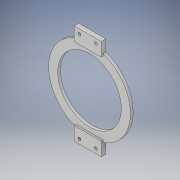
# Autodesk Inventor part: LED_Ring
Saved by Autodesk Inventor 2017 (Build 210142000, 142)
## iProperties
Part Number: LED_Ring
Material: Generisch
Document SubType Name: Modeling
Designer: Fabio
Density: 1 g/cm^3
Appearance: Vorgabe
Author: Fabio
Autodesk Inventor part; units mm, degrees
ref_plane "YZ Plane" through (0, 0, 0) normal (1, 0, 0) x (0, 1, 0)
ref_plane "XZ Plane" through (0, 0, 0) normal (0, 1, 0) x (-1, 0, 0)
ref_plane "XY Plane" through (0, 0, 0) normal (0, 0, 1) x (1, 0, 0)
sketch "Skizze1" plane through (0, 0, 0) normal (0, 1, 0) x (-1, 0, 0)
  circle A0 centre (0, 0) radius 45
  circle A1 centre (0, 0) radius 35
  dimension "d0" = 90
  dimension "d1" = 70
  constraints: 2 centre point, 2 coincident
  measures "d0" diameter of A0
  measures "d1" diameter of A1
extrude "Extrusion1" add sketch "Skizze1" along normal blind 3
sketch "Skizze4" plane through (0, 3, 0) normal (0, 1, 0) x (1, 0, 0)
  line L0 (0, 0) -> (0, -55) construction
  line L1 (0, -55) -> (-15, -55)
  line L2 (-15, -55) -> (-15, -40)
  circle A0 centre (0, 0) radius 35 projected
  line L3 (-15, -40) -> (0, -40)
  line L4 (0, -55) -> (15, -55)
  line L5 (15, -55) -> (15, -40)
  line L6 (15, -40) -> (0, -40)
  line L7 (0, 0) -> (-16.8776, 0) construction
  line L8 (0, 55) -> (-15, 55)
  line L9 (-15, 55) -> (-15, 40)
  line L10 (-15, 40) -> (0, 40)
  line L11 (0, 55) -> (15, 55)
  line L12 (15, 55) -> (15, 40)
  line L13 (15, 40) -> (0, 40)
  dimension "d28" = 15
  dimension "d29" = 15
  dimension "d30" = 40
  constraints: 28 end point, 8 symmetric about line, 2 horizontal, 2 perpendicular, 1 point on line, 1 vertical
  measures "d28" distance of L1.end L2.end
  measures "d29" distance of L0.end L1.end
  measures "d30" distance from line of L0.start L3
extrude "Extrusion3" add sketch "Skizze4" against normal blind 5 contours L1 L2 L3 L6 L5 L4 | L11 L12 L13 L10 L9 L8
sketch "Skizze5" plane through (0, 3, 0) normal (0, 1, 0) x (1, 0, 0)
  arc A0 (-15, 42.4264) -> (-15, -42.4264) centre (0, 0) ccw construction
  line L0 (15, -55) -> (-15, -55) construction
  arc A1 (15, -42.4264) -> (15, 42.4264) centre (0, 0) ccw construction
  line L1 (15, -42.4264) -> (15, -55) construction
  line L2 (-15, -55) -> (-15, -42.4264) construction
  line L3 (-15, -55) -> (-15, -40) construction
  line L4 (-15, -47.5) -> (15, -47.5) construction
  line L5 (15, -40) -> (15, -55) construction
  line L6 (0, 0) -> (20.9136, 0) construction
  point P0 (9, -50)
  point P1 (-9, -50)
  point P2 (9, 50)
  point P3 (-9, 50)
  dimension "d43" = 5
  dimension "d44" = 5
  dimension "d45" = 18
  dimension "d46" = 6
  constraints: 4 end point, 2 midpoint, 2 symmetric about line, 1 horizontal
  measures "d43" distance from line of point (9, -50) L0
  measures "d44" distance from line of L0 point (-9, -50)
  measures "d45" distance of point (-9, -50) point (9, -50)
  measures "d46" distance from line of L1 point (9, -50)
hole "Bohrung2" at (9, 3, 50) at (-9, 3, 50) at (9, 3, -50) at (-9, 3, -50) direction (0, -1, 0) diameter 3.3 depth 8 tip angle 118
